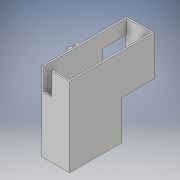
# Autodesk Inventor part: Part3
Saved by Autodesk Inventor 2019 (Build 230136000, 136)
## iProperties
Created: 2018-10-08
Part Number: Part3
Material: Generic
Document SubType Name: Modeling
Designer: Steven
Density: 1 g/cm^3
Appearance: Default
Author: Steven
Autodesk Inventor part; units mm, degrees
ref_plane "YZ Plane" through (0, 0, 0) normal (1, 0, 0) x (0, 1, 0)
ref_plane "XZ Plane" through (0, 0, 0) normal (0, 1, 0) x (-1, 0, 0)
ref_plane "XY Plane" through (0, 0, 0) normal (0, 0, 1) x (1, 0, 0)
sketch "Sketch1" plane through (0, 0, 0) normal (0, 1, 0) x (-1, 0, 0)
  line L0 (0, 0) -> (34, 0)
  line L1 (34, 0) -> (34, -104)
  line L2 (34, -104) -> (0, -104)
  line L3 (0, -104) -> (0, 0)
  dimension "d0" = 34
  dimension "d1" = 104
  constraints: 8 end point, 2 parallel, 1 horizontal, 1 perpendicular
  measures "d0" distance of L1.end L2.end
  measures "d1" distance of L0.end L1.end
extrude "Extrusion1" add sketch "Sketch1" along normal blind 2
sketch "Sketch2" plane through (0, 2, 0) normal (0, 1, 0) x (1, 0, 0)
  line L0 (-32, 2) -> (-2, 2)
  line L1 (-2, 2) -> (-2, 102)
  line L2 (-2, 102) -> (-32, 102)
  line L3 (-32, 102) -> (-32, 2)
  line L4 (-34, 0) -> (0, 0) projected
  line L5 (0, 104) -> (-34, 104) projected
  line L6 (-34, 104) -> (-34, 0) projected
  line L7 (0, 0) -> (0, 104) projected
  line L8 (-32, 2) -> (-2, 2)
  line L9 (-2, 2) -> (-2, 24)
  line L10 (-2, 24) -> (-32, 24)
  line L11 (-32, 24) -> (-32, 2)
  line L12 (-32, 24) -> (-2, 24)
  line L13 (-2, 24) -> (-2, 26.5)
  line L14 (-2, 26.5) -> (-32, 26.5)
  line L15 (-32, 26.5) -> (-32, 24)
  line L16 (-32, 26.5) -> (-2, 26.5)
  line L17 (-2, 26.5) -> (-2, 41.75)
  line L18 (-2, 41.75) -> (-32, 41.75)
  line L19 (-32, 41.75) -> (-32, 26.5)
  line L20 (-32, 41.75) -> (-2, 41.75)
  line L21 (-2, 41.75) -> (-2, 43.75)
  line L22 (-2, 43.75) -> (-32, 43.75)
  line L23 (-32, 43.75) -> (-32, 41.75)
  dimension "d4" = 2
  dimension "d5" = 2
  dimension "d6" = 2
  dimension "d7" = 2
  dimension "d8" = 30
  dimension "d9" = 22
  dimension "d10" = 30
  dimension "d11" = 2.5
  dimension "d12" = 30
  dimension "d13" = 15.25
  dimension "d14" = 30
  dimension "d15" = 2
  constraints: 40 end point, 10 parallel, 5 horizontal, 5 perpendicular
  measures "d4" distance between parallel lines of L4 L0
  measures "d5" distance between parallel lines of L5 L2
  measures "d6" distance between parallel lines of L6 L3
  measures "d7" distance between parallel lines of L7 L1
  measures "d8" distance of L10.end L9.end
  measures "d9" distance of L9.end L8.end
  measures "d10" distance of L14.end L13.end
  measures "d11" distance of L13.end L12.end
  measures "d12" distance of L18.end L17.end
  measures "d13" distance of L17.end L16.end
  measures "d14" distance of L22.end L21.end
  measures "d15" distance of L21.end L20.end
extrude "Extrusion2" add sketch "Sketch2" along normal blind 15 contours L3 L14 L1 L10 | L3 L22 L1 L18 | L6 L5 L7 L4
sketch "Sketch3" plane through (0, 17, 0) normal (0, 1, 0) x (1, 0, 0)
  line L0 (-34, 104) -> (0, 104) projected
  line L1 (0, 104) -> (0, 0) projected
  line L2 (-34, 104) -> (0, 104)
  line L3 (0, 104) -> (0, 0)
  line L4 (0, 0) -> (-34, 0)
  line L5 (-34, 0) -> (-34, 104)
  line L6 (-2, 2) -> (-32, 2) projected
  line L7 (-2, 102) -> (-2, 43.75) projected
  line L8 (-32, 2) -> (-2, 2)
  line L9 (-2, 2) -> (-2, 102)
  line L10 (-2, 102) -> (-32, 102)
  line L11 (-32, 102) -> (-32, 2)
  constraints: 16 end point, 4 parallel, 2 horizontal, 2 perpendicular
extrude "Extrusion3" add sketch "Sketch3" along normal blind 80
sketch "Sketch4" plane through (0, 0, 0) normal (0, -1, 0) x (1, 0, 0)
  line L0 (0, -104) -> (0, 0) projected
  line L1 (0, 0) -> (-34, 0)
  line L2 (-34, 0) -> (-34, -62)
  line L3 (-34, -62) -> (0, -62)
  line L4 (0, -62) -> (0, 0)
  line L5 (-34, -104) -> (0, -104) projected
  line L6 (0, -62) -> (-34, -62)
  line L7 (-34, -62) -> (-34, -104)
  line L8 (-34, -104) -> (0, -104)
  line L9 (0, -104) -> (0, -62)
  dimension "d20" = 34
  dimension "d21" = 62
  constraints: 16 end point, 4 parallel, 2 horizontal, 2 perpendicular
  measures "d20" distance of L3.end L2.end
  measures "d21" distance of L2.end L1.end
extrude "Extrusion4" cut sketch "Sketch4" against normal blind 50 contours L5 L7 L3 L0
sketch "Sketch5" plane through (0, 50, 0) normal (0, -1, 0) x (1, 0, 0)
  line L0 (-34, -62) -> (-32, -62) projected
  line L1 (0, 0) -> (0, -104) projected
  line L2 (-34, -62) -> (0, -62)
  line L3 (0, -62) -> (0, -104)
  line L4 (0, -104) -> (-34, -104)
  line L5 (-34, -104) -> (-34, -62)
  constraints: 8 end point, 2 parallel, 1 horizontal, 1 perpendicular
extrude "Extrusion5" add sketch "Sketch5" along normal blind 2
sketch "Sketch6" plane through (0, 0, -62) normal (0, 0, -1) x (-1, 0, 0)
  line L0 (0, 0) -> (0, 48) projected
  line L1 (34, 0) -> (0, 0) projected
  line L2 (0, 48) -> (34, 48)
  line L3 (34, 48) -> (34, 0)
  line L4 (34, 0) -> (0, 0)
  line L5 (0, 0) -> (0, 48)
  constraints: 8 end point, 2 parallel, 1 horizontal, 1 perpendicular
extrude "Extrusion6" add sketch "Sketch6" along normal blind 2
sketch "Sketch7" plane through (-34, 0, 0) normal (0, 0, 1) x (1, 0, 0)
  line L0 (0, 97) -> (34, 97) projected
  line L1 (2, 97) -> (12, 97)
  line L2 (12, 97) -> (12, 70)
  line L3 (12, 70) -> (2, 70)
  line L4 (2, 70) -> (2, 97)
  line L5 (34, 0) -> (0, 0) projected
  line L6 (0, 0) -> (0, 97) projected
  dimension "d28" = 70
  dimension "d29" = 2
  dimension "d30" = 10
  constraints: 8 end point, 2 parallel, 1 horizontal, 1 perpendicular, 1 point on line
  measures "d28" distance between parallel lines of L5 L3
  measures "d29" distance between parallel lines of L6 L4
  measures "d30" distance between parallel lines of L4 L2
extrude "Extrusion7" cut sketch "Sketch7" against normal blind 2
sketch "Sketch8" plane through (-34, 0, 0) normal (-1, 0, 0) x (0, 0, 1)
  line L0 (-102, 50) -> (-102, 97) projected
  line L1 (-102, 50) -> (-72, 50)
  line L2 (-72, 50) -> (-72, 80)
  line L3 (-72, 80) -> (-102, 80)
  line L4 (-102, 80) -> (-102, 50)
  point P0 (0, 0)
  dimension "d33" = 30
  dimension "d34" = 30
  constraints: 8 end point, 2 parallel, 1 horizontal, 1 perpendicular
  measures "d33" distance of L3.end L2.end
  measures "d34" distance of L2.end L1.end
extrude "Extrusion8" cut sketch "Sketch8" against normal blind 2
sketch "Sketch9" plane through (-34, 0, 0) normal (-1, 0, 0) x (0, 0, 1)
  line L0 (0, 0) -> (-64, 0) projected
  line L1 (-64, 0) -> (-59, 0)
  line L2 (-59, 0) -> (-59, 80)
  line L3 (-59, 80) -> (-64, 80)
  line L4 (-64, 80) -> (-64, 0)
  line L5 (-55.5, 0) -> (-50.5, 0)
  line L6 (-50.5, 0) -> (-50.5, 80)
  line L7 (-50.5, 80) -> (-55.5, 80)
  line L8 (-55.5, 80) -> (-55.5, 0)
  dimension "d37" = 5
  dimension "d38" = 80
  dimension "d39" = 5
  dimension "d40" = 80
  dimension "d41" = 3.5
  constraints: 16 end point, 4 parallel, 2 horizontal, 2 perpendicular, 1 point on line
  measures "d37" distance of L3.end L2.end
  measures "d38" distance of L2.end L1.end
  measures "d39" distance of L7.end L6.end
  measures "d40" distance of L6.end L5.end
  measures "d41" distance between parallel lines of L2 L8
extrude "Extrusion9" add sketch "Sketch9" along normal blind 20
sketch "Sketch10" plane through (-34, 0, -50.5) normal (0, 0, 1) x (1, 0, 0)
  line L0 (0, 80) -> (-20, 80) construction
  line L1 (-10, 80) -> (-10, 0) construction
  line L2 (34, 0) -> (-20, 0) construction
  circle A0 centre (-10, 60) radius 5
  circle A1 centre (-10, 70) radius 3
  circle A2 centre (-10, 50) radius 3
  circle A3 centre (-10, 10) radius 4.75
  dimension "d44" = 10
  dimension "d45" = 20
  dimension "d46" = 6
  dimension "d47" = 6
  dimension "d48" = 10
  dimension "d49" = 30
  dimension "d50" = 9.5
  dimension "d51" = 50
  constraints: 5 point on line, 4 centre point, 2 end point, 1 midpoint, 1 vertical
  measures "d44" diameter of A0
  measures "d45" distance from line of L0 A0.centre
  measures "d46" diameter of A1
  measures "d47" diameter of A2
  measures "d48" distance from line of L0 A1.centre
  measures "d49" distance from line of A2.centre L0
  measures "d50" diameter of A3
  measures "d51" distance of A0.centre A3.centre
extrude "Extrusion10" cut sketch "Sketch10" against normal blind 5
sketch "Sketch11" plane through (0, 0, -64) normal (0, 0, -1) x (-1, 0, 0)
  line L0 (34, 80) -> (54, 80) projected
  line L1 (44, 80) -> (44, 0) construction
  circle A0 centre (44, 70) radius 3 projected
  circle A1 centre (44, 70) radius 3
  circle A2 centre (44, 50) radius 3 projected
  circle A3 centre (44, 50) radius 3
  circle A4 centre (44, 10) radius 4.75 projected
  circle A5 centre (44, 10) radius 4.75
  line L2 (46.4853, 66) -> (50, 62.4853)
  line L3 (50, 62.4853) -> (50, 57.5147)
  line L4 (50, 57.5147) -> (46.4853, 54)
  line L5 (46.4853, 54) -> (41.5147, 54)
  line L6 (41.5147, 54) -> (38, 57.5147)
  line L7 (38, 57.5147) -> (38, 62.4853)
  line L8 (38, 62.4853) -> (41.5147, 66)
  line L9 (41.5147, 66) -> (46.4853, 66)
  line L10 (54, 0) -> (54, 80) projected
  line L11 (46.4853, 66) -> (54, 66)
  line L12 (54, 66) -> (54, 54)
  line L13 (54, 54) -> (46.4853, 54)
  line L14 (46.4853, 54) -> (46.4853, 66)
  point P0 (0, 0)
  point P1 (44, 60)
  point P2 (44, 60)
  point P3 (44, 66)
  constraints: 26 end point, 4 coincident, 3 centre point, 3 point on line, 2 midpoint, 2 parallel, 1 horizontal, 1 perpendicular, 1 vertical, 17 other
extrude "Extrusion11" cut sketch "Sketch11" against normal blind 5
body "Solid1"
